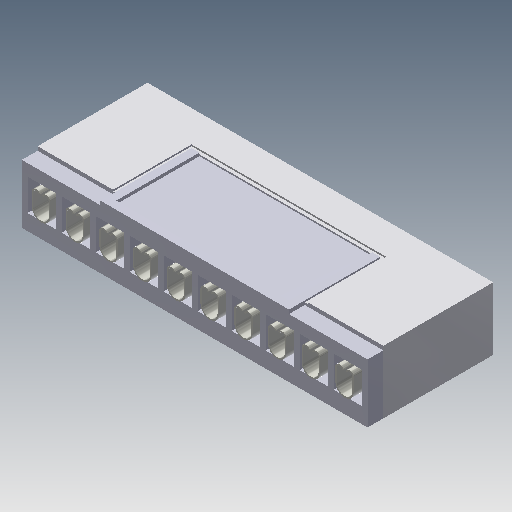
# Autodesk Inventor part: config - j9c2 connector
Saved by Autodesk Inventor 2020 (Build 240152000, 152)
## iProperties
Created: 2005-12-05
Part Number: config - j9c2 connector
Document SubType Name: Modeling
Designer: Simon.Ng@autodesk.com
Stock Number: config - j9c2 connector
Density: 1 g/cm^3
Material: Generic
Mass: 0.594326 g
Surface Area: 11.2983 cm^2
Volume: 0.594326 cm^3
Appearance: Cool White
Company: Autodesk Asia Pte. Ltd.
Title: PC Demo
Author: Simon.Ng@autodesk.com
Autodesk Inventor part; units mm, degrees
ref_plane "YZ Plane" through (0, 0, 0) normal (1, 0, 0) x (0, 1, 0)
ref_plane "XZ Plane" through (0, 0, 0) normal (0, 1, 0) x (-1, 0, 0)
sketch "Sketch1" plane through (0, 0, 0) normal (0, 0, 1) x (1, 0, 0)
  line L0 (0, 3.2) -> (0, -2.4) projected
  line L1 (-13.2, 0) -> (17.6, 0) projected
  line L2 (-11, 2) -> (11, 2)
  line L3 (11, 2) -> (11, -2)
  line L4 (11, -2) -> (-11, -2)
  line L5 (-11, -2) -> (-11, 2)
  dimension "d0" = 22
  dimension "d1" = 4
  constraints: 8 end point, 2 parallel, 1 horizontal, 1 perpendicular, 2 other
  measures "d0" distance of L2.start L2.end
  measures "d1" distance of L4.end L2.start
extrude "Extrusion1" add sketch "Sketch1" along normal blind 8
sketch "Sketch2" plane through (0, 0, 8) normal (0, 0, 1) x (1, 0, 0)
  line L0 (11, 2) -> (11, -2) projected
  line L1 (-13.2, 0) -> (17.6, 0) projected
  line L2 (10.6364, 1) -> (8.8364, 1)
  line L3 (8.8364, 1) -> (8.8364, -1)
  line L4 (8.8364, -1) -> (10.6364, -1)
  line L5 (10.6364, -1) -> (10.6364, 1)
  dimension "d4" = 2
  dimension "d5" = 1.8
  dimension "d6" = 0.3636
  constraints: 8 end point, 2 parallel, 1 horizontal, 1 perpendicular, 1 other
  measures "d4" distance of L4.end L2.start
  measures "d5" distance of L2.start L2.end
  measures "d6" distance between parallel lines of L0 L5
extrude "Extrusion2" cut sketch "Sketch2" against normal blind 3
pattern_linear "Rectangular Pattern1" count 10 spacing 2.1636 along (-1, 0, 0) of "Extrusion2"
sketch "Sketch3" plane through (0, 0, 8) normal (0, 0, 1) x (1, 0, 0)
  line L0 (-11, 2) -> (-6, 2)
  line L1 (-6, 2) -> (-6, 1.75)
  line L2 (-6, 1.75) -> (-11, 1.75)
  line L3 (-11, 1.75) -> (-11, 2)
  line L4 (11, 2) -> (6, 2)
  line L5 (6, 2) -> (6, 1.75)
  line L6 (6, 1.75) -> (11, 1.75)
  line L7 (11, 1.75) -> (11, 2)
  dimension "d12" = 5
  dimension "d13" = 0.25
  constraints: 16 end point, 4 parallel, 2 collinear, 2 horizontal, 2 perpendicular
  measures "d12" distance of L1.end L2.end
  measures "d13" distance of L0.end L1.end
extrude "Extrusion3" cut sketch "Sketch3" against normal blind 1
sketch "Sketch4" plane through (-11, 2, 0) normal (0, 1, 0) x (1, 0, 0)
  line L0 (0, -7) -> (5, -7) projected
  line L1 (5, -7) -> (4.8, -7)
  line L2 (4.8, -7) -> (4.8, -2)
  line L3 (4.8, -2) -> (5, -2)
  line L4 (5, -2) -> (5, -7)
  line L5 (17, -7) -> (17.2, -7)
  line L6 (17.2, -7) -> (17.2, -2)
  line L7 (17.2, -2) -> (17, -2)
  line L8 (17, -2) -> (17, -7)
  line L9 (17, -2) -> (17, -2.2)
  line L10 (5, -2.2) -> (5, -2)
  line L11 (5, -2) -> (17, -2)
  line L12 (17, -2) -> (17, -2.2)
  line L13 (17, -2.2) -> (5, -2.2)
  line L14 (5, -2.2) -> (5, -2)
  dimension "d16" = 0.2
  dimension "d19" = 5
  dimension "d20" = 0.2
  constraints: 28 end point, 7 parallel, 3 horizontal, 3 perpendicular, 2 equal length, 2 point on line
  measures "d16" distance of L2.end L3.end
  measures "d19" distance between parallel lines of L0 L3
  measures "d20" distance between parallel lines of L11 L13
extrude "Extrusion4" cut sketch "Sketch4" against normal blind 0.1
ref_plane "Work Plane1" through (0, 0, 7) normal (0, 0, 1) x (1, 0, 0)
split_face "Split1"
sketch "Sketch5" plane through (-6, 2, 8) normal (0, 1, 0) x (1, 0, 0)
  line L0 (12, 0) -> (12, 5.8) projected
  line L1 (12, 5.8) -> (0, 5.8) projected
  line L2 (0, 5.8) -> (0, 0) projected
  line L3 (0, 0) -> (12, 0) projected
  line L4 (0.5, 5.8) -> (11.5, 5.8)
  line L5 (11.5, 5.8) -> (11.5, 0.5)
  line L6 (11.5, 0.5) -> (0.5, 0.5)
  line L7 (0.5, 0.5) -> (0.5, 5.8)
  dimension "d24" = 0.5
  dimension "d25" = 0.5
  dimension "d26" = 0.5
  constraints: 8 end point, 2 parallel, 1 horizontal, 1 perpendicular, 1 point on line
  measures "d24" distance between parallel lines of L2 L7
  measures "d25" distance between parallel lines of L0 L5
  measures "d26" distance between parallel lines of L3 L6
extrude "Extrusion5" cut sketch "Sketch5" against normal blind 0.2 contours L5 L6 L7 L1
sketch "Sketch6" plane through (0, 0, 5) normal (0, 0, 1) x (1, 0, 0)
  line L0 (8.8364, -1) -> (10.6364, -1) construction
  line L1 (10.6364, 1) -> (8.8364, 1) construction
  line L2 (9.7364, 1) -> (9.7364, -1) construction
  arc A0 (10.3238, 0.5776) -> (9.7981, 0.6233) centre (10.053, 0.5091) ccw
  line L3 (10.3238, 0.5776) -> (10.3238, -0.3057)
  arc A1 (9.6746, 0.6233) -> (9.1489, 0.5776) centre (9.4197, 0.5091) ccw
  line L4 (9.1489, 0.5776) -> (9.1489, -0.3057)
  arc A2 (9.1489, -0.3057) -> (10.3238, -0.3057) centre (9.7364, -0.3057) ccw
  arc A3 (10.2364, 0.5656) -> (9.878, 0.5875) centre (10.053, 0.5091) ccw
  line L5 (10.2364, 0.5656) -> (10.2364, -0.3057)
  arc A4 (9.2364, -0.3057) -> (10.2364, -0.3057) centre (9.7364, -0.3057) ccw
  line L6 (9.2364, -0.3057) -> (9.2364, 0.5656)
  arc A5 (9.5948, 0.5875) -> (9.2364, 0.5656) centre (9.4197, 0.5091) ccw
  line L7 (9.5948, 0.5875) -> (9.6746, 0.6233)
  line L8 (9.878, 0.5875) -> (9.7981, 0.6233)
  dimension "d29" = 0.5
  constraints: 14 end point, 12 point on circle, 6 centre point, 4 symmetric about line, 2 midpoint, 2 tangent, 1 parallel, 5 other
  measures "d29" radius of A4
extrude "Extrusion6" add sketch "Sketch6" along normal blind 3.2
pattern_linear "Rectangular Pattern2" count 10 spacing 2.146 along (-1, 0, 0) of "Extrusion6"
equation "\"d20\" = d16"
equation "\"d25\" = d24"
equation "\"d26\" = d24"
body "Solid1"
